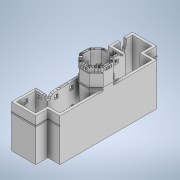
# Autodesk Inventor part: Part1
Saved by Autodesk Inventor 2020 (Build 240168000, 168)
## iProperties
Created: 2021-05-09
Part Number: Part1
Material: Generic
Document SubType Name: Modeling
Designer: Vlasciar
Density: 1 g/cm^3
Appearance: Default
Author: Vlasciar
Autodesk Inventor part; units mm, degrees
ref_plane "YZ Plane" through (0, 0, 0) normal (1, 0, 0) x (0, 1, 0)
ref_plane "XZ Plane" through (0, 0, 0) normal (0, 1, 0) x (-1, 0, 0)
ref_plane "XY Plane" through (0, 0, 0) normal (0, 0, 1) x (1, 0, 0)
sketch "Sketch1" plane through (0, 0, 0) normal (0, 1, 0) x (-1, 0, 0)
  line L0 (-10, -40) -> (10, -40)
  line L1 (10, -40) -> (10, 40)
  line L2 (10, 40) -> (-10, 40)
  line L3 (-10, 40) -> (-10, -40)
  line L4 (-10, -40) -> (10, 40) construction
  line L5 (10, -40) -> (-10, 40) construction
  line L6 (0, 30) -> (20, 30)
  line L7 (20, 30) -> (20, 50)
  line L8 (20, 50) -> (0, 50)
  line L9 (0, 50) -> (0, 30)
  line L10 (0, 30) -> (20, 50) construction
  line L11 (20, 30) -> (0, 50) construction
  line L12 (0, -50) -> (20, -50)
  line L13 (20, -50) -> (20, -30)
  line L14 (20, -30) -> (0, -30)
  line L15 (0, -30) -> (0, -50)
  line L16 (0, -50) -> (20, -30) construction
  line L17 (20, -50) -> (0, -30) construction
  line L18 (10, 4.1421) -> (10, -4.1421)
  line L19 (10, -4.1421) -> (4.1421, -10)
  line L20 (4.1421, -10) -> (-4.1421, -10)
  line L21 (-4.1421, -10) -> (-10, -4.1421)
  line L22 (-10, -4.1421) -> (-10, 4.1421)
  line L23 (-10, 4.1421) -> (-4.1421, 10)
  line L24 (-4.1421, 10) -> (4.1421, 10)
  line L25 (4.1421, 10) -> (10, 4.1421)
  point P0 (0, 0)
  point P1 (0, 0)
  point P2 (10, -40)
  point P3 (0, 40)
  point P4 (0, -40)
  point P5 (10, -30)
  point P6 (10, 30)
  point P7 (-10, -4.1421)
  dimension "d0" = 80
  dimension "d1" = 20
  dimension "d2" = 20
  dimension "d3" = 20
  constraints: 52 end point, 7 midpoint, 6 parallel, 5 perpendicular, 3 horizontal, 1 coincident, 1 point on line, 1 vertical alignment, 17 other
  measures "d0" distance of L0.end L1.end
  measures "d1" distance of L1.end L2.end
  measures "d2" distance of L8.end L7.end
  measures "d3" distance of L14.end L13.end
extrude "Extrusion1" add sketch "Sketch1" along normal blind 32
shell "Shell1" thickness 2 removed faces 1 at (3.3333, 32, 10)
extrude "Extrusion2" add sketch "Sketch1" along normal blind 47 contours L3 L23 L24 L25 L1 L19 L20 L21
sketch "Sketch2" plane through (-20, 0, -50) normal (-1, 0, 0) x (0, 0, 1)
  line L0 (0, 0) -> (20, 0) projected
  line L1 (8, 22) -> (11.5, 22)
  line L2 (11.5, 22) -> (11.5, 12)
  line L3 (11.5, 12) -> (8, 12)
  line L4 (8, 12) -> (8, 22)
  arc A0 (11.5, 22) -> (8, 22) centre (9.75, 17.3163) ccw
  line L5 (12.25, 12) -> (7.25, 12)
  line L6 (7.25, 12) -> (7.25, 22.5633)
  line L7 (12.25, 22.5633) -> (12.25, 12)
  arc A1 (12.25, 22.5633) -> (7.25, 22.5633) centre (9.75, 18.8216) ccw
  line L8 (8.5858, 23.1684) -> (8.5858, 24)
  line L9 (8.5858, 24) -> (9, 24)
  line L10 (9, 24) -> (8, 26)
  line L11 (8, 26) -> (8, 27.1645)
  line L12 (8, 27.1645) -> (7.25, 28.1134)
  line L13 (7.25, 28.1134) -> (7, 32)
  line L14 (12, 32) -> (43.8579, 32) projected
  line L15 (10.6101, 24) -> (10.3293, 23.2842)
  line L16 (7, 32) -> (11.5, 32)
  line L17 (11.5, 32) -> (12.167, 32)
  line L18 (45.8579, 32) -> (10, 32) projected
  line L19 (12.167, 32) -> (12.167, 28.6709)
  line L20 (12, 2) -> (12, 32) projected
  line L21 (12.167, 28.6709) -> (11.5, 27.1645)
  line L22 (11.5, 27.1645) -> (11.3101, 25.7841)
  line L23 (11.3101, 25.7841) -> (10.6101, 24)
  point P0 (50, 0)
  point P1 (12.6775, 32)
  point P2 (8, 12)
  point P3 (11.5, 12)
  point P4 (10.6101, 24)
  point P5 (12, 28.2938)
  dimension "d9" = 12
  dimension "d10" = 10
  dimension "d11" = 3.5
  dimension "d12" = 5
  dimension "d13" = 0.75
  dimension "d14" = 0.75
  dimension "d15" = 4.5
  constraints: 40 end point, 6 point on circle, 5 parallel, 4 point on line, 2 centre point, 2 horizontal, 2 perpendicular, 1 vertical
  measures "d9" distance between parallel lines of L0 L3
  measures "d10" distance of L3.end L1.start
  measures "d11" distance of L2.end L3.end
  measures "d12" radius of A0
  measures "d13" distance between parallel lines of L7 L2
  measures "d14" distance between parallel lines of L6 L4
  measures "d15" radius of A1
extrude "Extrusion3" cut sketch "Sketch2" against normal blind 2 contours A0 L1 | L1 L2 L3 L4
extrude "Extrusion4" cut sketch "Sketch2" against normal blind 1 contours L4 L5 L6 A1 L20 L2 A0 | L20 A1 L7 L5
extrude "Extrusion6" cut sketch "Sketch2" against normal blind 2 contours L8 L9 L10 L11 L12 L13 L16 L17 L20 L21 L22 L23 L15 A1
sketch "Sketch3" plane through (-20, 0, -50) normal (-1, 0, 0) x (0, 0, 1)
  line L0 (0, 0) -> (0, 32) projected
  line L1 (0, 0) -> (20, 0) projected
  line L2 (20, 0) -> (20, 32) projected
  line L3 (11.5, 27.1645) -> (11.3101, 25.7841) projected
  line L4 (11.3101, 25.7841) -> (10.3293, 23.2842) projected
  line L5 (9, 24) -> (8, 26) projected
  line L6 (0, 0) -> (0, 32) projected
  line L7 (0, 25) -> (20, 25)
  line L8 (20, 0) -> (20, 32) projected
  line L9 (0, 26) -> (20, 26)
  point P0 (50, 0)
  point P1 (11.3398, 26)
  point P2 (11.0025, 25)
  point P3 (0, 26)
  point P4 (0, 25)
  point P5 (8.5, 25)
  dimension "d24" = 25
  dimension "d25" = 1
  constraints: 4 end point, 4 point on line, 1 horizontal, 1 perpendicular
  measures "d24" distance between parallel lines of L1 L7
  measures "d25" distance between parallel lines of L9 L7
extrude "Extrusion7" add sketch "Sketch3" along normal blind 0.25 contours L0 L9 L5 L7 | L7 L4 L3 L9 L2
ref_plane "Work Plane1" through (-20.25, 25, -50) normal (0, 1, 0) x (0, 0, 1)
sketch "Sketch4" plane through (-20.25, 25, -50) normal (0, 1, 0) x (0, 0, 1)
  line L0 (20.25, 0) -> (20.25, 10)
  line L1 (20.25, 10) -> (79.75, 10)
  line L2 (79.75, 10) -> (79.75, 0)
  line L3 (79.75, 0) -> (100.25, 0)
  line L4 (100.25, 0) -> (100.25, 20.5)
  line L5 (100.25, 20.5) -> (90.25, 20.5)
  line L6 (90.25, 20.5) -> (90.25, 30.25)
  line L7 (9.75, 30.25) -> (9.75, 20.5)
  line L8 (9.75, 20.5) -> (-0.25, 20.5)
  line L9 (-0.25, 20.5) -> (-0.25, 0)
  line L10 (8, 0) -> (0, 0) projected
  line L11 (-0.25, 0) -> (0, 0)
  line L12 (0, 20.25) -> (0, 0.25) projected
  line L13 (10, 20.25) -> (0, 20.25) projected
  line L14 (10, 30.25) -> (10, 20.25) projected
  line L15 (9.75, 30.25) -> (10, 30.25)
  line L16 (90, 20.25) -> (90, 30.25) projected
  line L17 (90, 30.25) -> (10, 30.25) projected
  line L18 (90, 30.25) -> (90.25, 30.25)
  line L19 (100, 0.25) -> (100, 20.25) projected
  line L20 (80, 10.25) -> (80, 0.25) projected
  line L21 (54.1421, 10.25) -> (80, 10.25) projected
  line L22 (20, 0.25) -> (20, 10.25) projected
  line L23 (20, 0.25) -> (20, 0) projected
  line L24 (20.25, 0) -> (20, 0)
  line L25 (0, 0) -> (20.25, 0)
  line L26 (10, 30.25) -> (90, 30.25)
  line L27 (90, 30.25) -> (90, 20.25)
  line L28 (100, 20.25) -> (90, 20.25)
  line L29 (100, 20.25) -> (100, 0.25)
  line L30 (100, 0.25) -> (80, 0.25)
  line L31 (20, 10.25) -> (80, 10.25) projected
  line L32 (80, 10.25) -> (80, 0.25) projected
  line L33 (80, 10.25) -> (80, 0.25)
  line L34 (80, 10.25) -> (20, 10.25)
  line L35 (20, 10.25) -> (20, 0)
  line L36 (20, 0.25) -> (11.0025, 0.25) projected
  line L37 (0, 0.25) -> (0, 0)
  point P0 (50, 20.25)
  dimension "d28" = 0.25
  dimension "d29" = 0.25
  dimension "d30" = 0.25
  dimension "d31" = 0.25
  dimension "d32" = 0.25
  dimension "d33" = 0.25
  dimension "d34" = 0.25
  dimension "d35" = 0.25
  constraints: 48 end point, 9 perpendicular, 4 collinear, 3 horizontal, 2 point on line, 2 vertical, 1 parallel
  measures "d28" distance between parallel lines of L12 L9
  measures "d29" distance between parallel lines of L13 L8
  measures "d30" distance between parallel lines of L14 L7
  measures "d31" distance between parallel lines of L6 L16
  measures "d32" distance between parallel lines of L4 L19
  measures "d33" distance between parallel lines of L20 L2
  measures "d34" distance between parallel lines of L21 L1
  measures "d35" distance between parallel lines of L22 L0
extrude "Extrusion8" add sketch "Sketch4" along normal blind 1 contours L24 L23 L22 L31 L21 L20 L30 L19 L28 L16 L18 L6 L5 L4 L3 L2 L1 L0
extrude "Extrusion9" add sketch "Sketch4" along normal blind 1 contours L11 L9 L8 L7 L15 L14 L13 L12 L37
sketch "Sketch5" plane through (0, 32, 0) normal (0, 1, 0) x (1, 0, 0)
  line L0 (-10, 30) -> (-10, 4.1421) projected
  line L1 (-10, 4.1421) -> (-8, 6.1421) projected
  line L2 (-8, 6.1421) -> (-8, 32) projected
  line L3 (-10, 30) -> (-8, 30)
  line L4 (-8, 32) -> (-8, 6.1421) projected
  line L5 (-10, 30) -> (-10, -30) projected
  line L6 (-10, -30) -> (-8, -30)
  line L7 (-8, -6.1421) -> (-8, -32) projected
  line L8 (-8, -30) -> (-8, -6.1421)
  line L9 (-10, -4.1421) -> (-4.1421, -10) projected
  line L10 (-10, -4.1421) -> (-10, -30)
  line L11 (-8, -6.1421) -> (-10, -4.1421)
  point P0 (0, 0)
  constraints: 10 end point, 2 parallel, 2 point on line, 1 horizontal, 1 vertical
extrude "Extrusion10" add sketch "Sketch5" along normal blind 2.5
sketch "Sketch6" plane through (-10, 47, -4.1421) normal (-1, 0, 0) x (0, 0, 1)
  line L0 (-25.8579, -47) -> (34.1421, -47) projected
  line L1 (6.0171, -18.8839) -> (2.2671, -18.8839)
  line L2 (2.2671, -18.8839) -> (2.2671, -14.3839)
  line L3 (2.2671, -14.3839) -> (6.0171, -14.3839)
  line L4 (6.0171, -14.3839) -> (6.0171, -18.8839)
  line L5 (6.0171, -18.8839) -> (2.2671, -14.3839) construction
  line L6 (2.2671, -18.8839) -> (6.0171, -14.3839) construction
  line L7 (5.5171, -18.2839) -> (2.7671, -18.2839)
  line L8 (2.7671, -18.2839) -> (2.7671, -14.9839)
  line L9 (2.7671, -14.9839) -> (5.5171, -14.9839)
  line L10 (5.5171, -14.9839) -> (5.5171, -18.2839)
  line L11 (5.5171, -18.2839) -> (2.7671, -14.9839) construction
  line L12 (2.7671, -18.2839) -> (5.5171, -14.9839) construction
  point P0 (4.1421, -47)
  point P1 (4.1421, -16.6339)
  point P2 (4.1421, -47)
  dimension "d42" = 3.75
  dimension "d43" = 4.5
  dimension "d44" = 2.75
  constraints: 24 end point, 5 midpoint, 4 parallel, 2 horizontal, 2 perpendicular, 1 point on line, 1 vertical alignment
  measures "d42" distance of L2.end L3.end
  measures "d43" distance of L1.end L2.end
  measures "d44" distance of L8.end L9.end
extrude "Extrusion11" cut sketch "Sketch6" against normal blind 2.5 contours L7 L8 L9 L10
extrude "Extrusion12" cut sketch "Sketch6" against normal blind 0.5 contours L1 L2 L3 L4 | L7 L8 L9 L10
pattern_linear "Rectangular Pattern1" count 3 spacing 12.5 along (0, 0, 1) count 2 spacing 14 along (0, -1, 0) of "Extrusion12", "Extrusion11"
pattern_linear "Rectangular Pattern2" count 3 spacing 12.5 along (0, 0, -1) count 2 spacing 14 along (0, -1, 0) of "Extrusion12", "Extrusion11"
sketch "Sketch7" plane through (-10, 47, -4.1421) normal (-1, 0, 0) x (0, 0, 1)
  line L0 (-25.8579, -12.5) -> (0, -12.5) projected
  line L1 (-25.8579, -15) -> (-25.8579, -12.5) projected
  line L2 (-25.8579, -15) -> (-24.9155, -14.8512)
  line L3 (-24.9155, -14.8512) -> (-24.7999, -14.2836)
  line L4 (-24.7999, -14.2836) -> (-23.2973, -13.787)
  line L5 (-23.2973, -13.787) -> (-22.7637, -12.9023)
  line L6 (-22.7637, -12.9023) -> (-22.5613, -12.5)
  line L7 (-22.5613, -12.5) -> (-19.8497, -12.5)
  line L8 (-19.8497, -12.5) -> (-17.8318, -13.1696)
  line L9 (-13.0388, -13.2248) -> (-11.5153, -12.5)
  line L10 (-11.5153, -12.5) -> (-9.0025, -12.5874)
  line L11 (-9.0025, -12.5874) -> (-6.8279, -12.5)
  line L12 (-6.8279, -12.5) -> (-5.8631, -12.6965)
  line L13 (-2.1188, -13.2003) -> (-1.5625, -13.178)
  line L14 (-1.5625, -13.178) -> (-0.4501, -12.6488)
  line L15 (-0.4501, -12.6488) -> (0, -12.5)
  line L16 (-17.8318, -13.1696) -> (-15.3761, -13.3447)
  line L17 (-15.3761, -13.3447) -> (-12.9874, -13.2003)
  line L18 (-5.8631, -12.6965) -> (-3.9239, -12.8348)
  line L19 (-3.9239, -12.8348) -> (-2.1188, -13.2003)
  point P0 (4.1421, -47)
  constraints: 36 end point, 7 point on line, 4 parallel
extrude "Extrusion13" cut sketch "Sketch7" against normal up to surface (2 mm away)
pattern_linear "Rectangular Pattern3" count 2 spacing 9 along (0, 1, 0) of "Extrusion11", "Extrusion12"
sketch "Sketch8" plane through (0, 47, 0) normal (0, 1, 0) x (1, 0, 0)
  line L0 (10, -4.1421) -> (10, 4.1421) projected
  line L1 (8, 3.3137) -> (8, -3.3137)
  line L2 (8, -3.3137) -> (3.3137, -8)
  line L3 (3.3137, -8) -> (-3.3137, -8)
  line L4 (-3.3137, -8) -> (-8, -3.3137)
  line L5 (-8, -3.3137) -> (-8, 3.3137)
  line L6 (-8, 3.3137) -> (-3.3137, 8)
  line L7 (-3.3137, 8) -> (3.3137, 8)
  line L8 (3.3137, 8) -> (8, 3.3137)
  point P0 (0, 0)
  point P1 (0, 0)
  dimension "d66" = 2
  dimension "d67" = 2
  constraints: 16 end point, 1 coincident, 17 other
  measures "d66" distance from line of L0 L1.start
  measures "d67" distance from line of L0 L1.end
extrude "Extrusion14" cut sketch "Sketch8" against normal blind 45
sketch "Sketch9" plane through (-10, 47, -4.1421) normal (-1, 0, 0) x (0, 0, 1)
  line L0 (8.2843, -12.5) -> (34.1421, -12.5) projected
  line L1 (8.2843, -12.5) -> (8.2843, 0) projected
  line L2 (0, -12.5) -> (0, 0) projected
  line L3 (8.2843, -12.5) -> (10.2843, -12.5) projected
  line L4 (8.4943, -12.5) -> (-0.21, -12.5)
  line L5 (-0.21, -12.5) -> (-0.21, -11.5)
  line L6 (-0.21, -11.5) -> (8.4943, -11.5)
  line L7 (8.4943, -11.5) -> (8.4943, -12.5)
  line L8 (-0.21, -12.1053) -> (8.4943, -12.1053)
  line L9 (8.4943, -12.1053) -> (8.4292, -12.1053)
  line L10 (8.4943, -12.5) -> (8.2843, -12.5)
  line L11 (8.2843, -12.5) -> (8.2843, -12.1053)
  line L12 (8.2843, -12.1053) -> (8.4943, -12.1053)
  line L13 (8.4943, -12.1053) -> (8.4943, -12.5)
  point P0 (4.1421, -47)
  point P1 (8.2843, -12.5)
  dimension "d70" = 0.21
  dimension "d71" = 0.21
  dimension "d72" = 1
  constraints: 20 end point, 6 point on line, 4 parallel, 3 perpendicular, 2 horizontal
  measures "d70" distance between parallel lines of L2 L5
  measures "d71" distance between parallel lines of L7 L1
  measures "d72" distance between parallel lines of L6 L4
extrude "Extrusion15" add sketch "Sketch9" along normal blind 0.5
pattern_circular "Circular Pattern1" count 8 over 360 about axis through (0, -10, 0) along (0, 1, 0) of "Extrusion15"
pattern_linear "Rectangular Pattern4" count 2 spacing 9 along (0, 1, 0) of "Extrusion15", "Circular Pattern1"
sketch "Sketch10" plane through (-10, 47, -4.1421) normal (-1, 0, 0) x (0, 0, 1)
  line L0 (0, -2.5) -> (8.2843, -2.5) projected
  line L1 (0, 0) -> (8.2843, 0) projected
  line L2 (7.4558, 0) -> (0.8284, 0) projected
  line L3 (4.9026, -2.5) -> (3.3817, -2.5)
  line L4 (3.3817, -2.5) -> (3.3817, -0.5122)
  line L5 (4.9026, -0.5122) -> (4.9026, -2.5)
  arc A0 (4.9026, -0.5122) -> (3.3817, -0.5122) centre (4.1421, -1.1616) ccw
  arc A1 (6.9026, -0.5122) -> (5.3817, -0.5122) centre (6.1421, -1.1616) ccw
  line L6 (6.9026, -0.5122) -> (6.9026, -2.5)
  line L7 (5.3817, -2.5) -> (5.3817, -0.5122)
  line L8 (6.9026, -2.5) -> (5.3817, -2.5)
  arc A2 (2.9026, -0.5122) -> (1.3817, -0.5122) centre (2.1421, -1.1616) ccw
  line L9 (2.9026, -0.5122) -> (2.9026, -2.5)
  line L10 (2.9026, -2.5) -> (1.3817, -2.5)
  line L11 (1.3817, -2.5) -> (1.3817, -0.5122)
  point P0 (4.1421, -47)
  point P1 (4.1421, -1.25)
  dimension "d81" = 1
  dimension "d84" = 2
  dimension "d91" = 2
  constraints: 18 end point, 6 point on circle, 3 centre point, 3 horizontal, 1 parallel, 1 perpendicular, 18 other
  measures "d81" radius of A0
  measures "d84" distance of A0.centre A1.centre
  measures "d91" distance of A0.centre A2.centre
extrude "Extrusion16" cut sketch "Sketch10" against normal blind 0.5
pattern_circular "Circular Pattern2" count 8 over 360 about axis through (0, -10, 0) along (0, 1, 0) of "Extrusion16"
sketch "Sketch11" plane through (0, 47, 0) normal (0, 1, 0) x (1, 0, 0)
  line L0 (-8, 3.3137) -> (-3.3137, 8) projected
  line L1 (-3.3137, 8) -> (3.3137, 8) projected
  line L2 (3.3137, 8) -> (8, 3.3137) projected
  line L3 (8, 3.3137) -> (8, -3.3137) projected
  line L4 (8, -3.3137) -> (3.3137, -8) projected
  line L5 (3.3137, -8) -> (-3.3137, -8) projected
  line L6 (-3.3137, -8) -> (-8, -3.3137) projected
  line L7 (-8, -3.3137) -> (-8, 3.3137) projected
  line L8 (-4.1421, 10) -> (-10, 4.1421) projected
  line L9 (-10, 4.1421) -> (-10, -4.1421) projected
  line L10 (-10, -4.1421) -> (-4.1421, -10) projected
  line L11 (-4.1421, -10) -> (4.1421, -10) projected
  line L12 (4.1421, -10) -> (10, -4.1421) projected
  line L13 (10, -4.1421) -> (10, 4.1421) projected
  line L14 (10, 4.1421) -> (4.1421, 10) projected
  line L15 (4.1421, 10) -> (-4.1421, 10) projected
  point P0 (0, 0)
extrude "Extrusion17" add sketch "Sketch11" along normal blind 1
sketch "Sketch12" plane through (-10, 44.5, 2.7605) normal (-1, 0, 0) x (0, 0, 1)
  line L0 (1.3817, 0) -> (1.3817, 3.5) projected
  line L1 (-6.9026, 3.5) -> (1.3817, 3.5) projected
  line L2 (-6.9026, 0) -> (-6.9026, 3.5) projected
  line L3 (1.3817, 0) -> (1.3817, 3.5) projected
  line L4 (1.3817, 3.0258) -> (-6.9026, 3.0258)
  line L5 (1.3817, 3.0258) -> (0.7961, 3.2794)
  line L6 (0.7961, 3.2794) -> (0.4566, 3.2083)
  line L7 (0.4566, 3.2083) -> (0.2925, 3.2794)
  line L8 (0.2925, 3.2794) -> (-0.1751, 3.3426)
  line L9 (-0.1751, 3.3426) -> (-0.2698, 3.2794)
  line L10 (-0.2698, 3.2794) -> (-0.5516, 3.2204)
  line L11 (-0.5516, 3.2204) -> (-1.0436, 3.2204)
  line L12 (-1.0436, 3.2204) -> (-1.3256, 3.3426)
  line L13 (-1.3256, 3.3426) -> (-1.5269, 3.2083)
  line L14 (-1.5269, 3.2083) -> (-1.8368, 3.3426)
  line L15 (-1.8368, 3.3426) -> (-2.2547, 3.399)
  line L16 (-2.2547, 3.399) -> (-2.628, 3.4494)
  line L17 (-2.628, 3.4494) -> (-2.9564, 3.3976)
  line L18 (-2.9564, 3.3976) -> (-3.395, 3.2204)
  line L19 (-3.395, 3.2204) -> (-3.8024, 3.2755)
  line L20 (-3.8024, 3.2755) -> (-4.2992, 3.3426)
  line L21 (-4.2992, 3.3426) -> (-4.7605, 3.3426)
  line L22 (-6.0742, 3.5) -> (0.5532, 3.5) projected
  line L23 (-4.7605, 3.3426) -> (-5.289, 3.2319)
  line L24 (-5.289, 3.2319) -> (-5.6985, 3.2873)
  line L25 (-5.6985, 3.2873) -> (-6.4207, 3.2204)
  line L26 (-6.4207, 3.2204) -> (-6.9026, 3.0258)
  point P0 (-2.7605, -44.5)
  constraints: 44 end point, 12 parallel, 6 point on line, 1 horizontal
extrude "Extrusion18" cut sketch "Sketch12" against normal blind 2 contours L5 L6 L7 L8 L9 L10 L11 L12 L13 L14 L15 L16 L17 L18 L19 L20 L21 L23 L24 L25 L26 L2 L1 L0
pattern_circular "Circular Pattern3" count 8 over 360 about axis through (0, -10, 0) along (0, 1, 0) of "Extrusion18"
sketch "Sketch13" plane through (-10, 35.5, -4.1421) normal (-1, 0, 0) x (0, 0, 1)
  line L0 (8.2843, 8) -> (0, 8) projected
  line L1 (0, 0) -> (0, 8) projected
  line L2 (8.2843, 0) -> (8.2843, 8) projected
  line L3 (2.2671, 1.6161) -> (2.2671, 6.1161) projected
  line L4 (2.2671, 6.1161) -> (6.0171, 6.1161) projected
  line L5 (6.0171, 6.1161) -> (6.0171, 1.6161) projected
  line L6 (1.9172, 6.1161) -> (6.3671, 6.1161)
  line L7 (6.3671, 6.1161) -> (4.1343, 8)
  line L8 (1.9172, 6.1161) -> (4.1343, 8)
  line L9 (1.9172, 6.1161) -> (6.3671, 6.1161)
  line L10 (6.3671, 6.1161) -> (4.1343, 8)
  line L11 (1.9172, 6.1161) -> (4.1343, 8)
  line L12 (6.0408, 6.2532) -> (4.1343, 7.8617)
  line L13 (2.2412, 6.2532) -> (6.0408, 6.2532)
  line L14 (2.2412, 6.2532) -> (4.1343, 7.8617)
  point P0 (4.1421, -35.5)
  point P1 (2.2671, 6.1161)
  point P2 (6.0171, 6.1161)
  dimension "d108" = 0.3499
  dimension "d109" = 0.35
  dimension "d110" = 4.15
  dimension "d111" = 4.1343
  constraints: 18 end point, 2 point on line, 1 horizontal
  measures "d108" distance from line of L3 L6.start
  measures "d109" distance from line of L5 L6.end
  measures "d110" distance from line of L7.end L2
  measures "d111" distance from line of L1 L7.end
extrude "Extrusion19" add sketch "Sketch13" along normal blind 0.5 contours L6 L8 L7 L4 | L13 L14 L12
extrude "Extrusion20" cut sketch "Sketch9" along normal blind 0.5 contours L1 L8 L7 L0 | L4 L2 L8 L1 | L4 L5 L8 L2
extrude "Extrusion21" add sketch "Sketch9" along normal blind 0.25 contours L1 L8 L7 L0 | L4 L2 L8 L1 | L4 L5 L8 L2
pattern_circular "Circular Pattern4" count 8 over 360 about axis through (0, -10, 0) along (0, 1, 0) of "Extrusion21", "Extrusion20"
pattern_linear "Rectangular Pattern5" count 2 spacing 9 along (0, 1, 0) of "Extrusion20", "Extrusion21", "Circular Pattern4"
extrude "Extrusion22" cut sketch "Sketch13" along normal blind 5 contours L13 L14 L12
extrude "Extrusion23" add sketch "Sketch13" along normal blind 0.25 contours L13 L14 L12
pattern_linear "Rectangular Pattern6" count 2 spacing 9 along (0, -1, 0) of "Extrusion22", "Extrusion23", "Extrusion19"
pattern_linear "Rectangular Pattern7" count 2 spacing 23 along (0, -1, 0) of "Extrusion23", "Extrusion22", "Extrusion19"
sketch "Sketch14" plane through (-10, 0, -30) normal (-1, 0, 0) x (0, 0, 1)
  line L0 (30, 0) -> (25.5, 0)
  line L1 (25.5, 0) -> (25.5, 9)
  line L2 (25.5, 9) -> (30, 9)
  line L3 (30, 9) -> (30, 0)
  arc A0 (30, 9) -> (25.5, 5.0081) centre (30.4006, 4.0161) ccw
  line L4 (60, 0) -> (0, 0)
  line L5 (34.5, 0) -> (34.5, 9)
  line L6 (34.5, 9) -> (30, 9)
  arc A1 (34.5, 5.0081) -> (30, 9) centre (29.5994, 4.0161) ccw
  line L7 (25.5, 0) -> (24.5, 0)
  line L8 (24.5, 0) -> (24.5, 9)
  line L9 (24.5, 9) -> (25.5, 9)
  line L10 (25.5, 9) -> (25.5, 0)
  line L11 (34.5, 0) -> (35.5, 0)
  line L12 (35.5, 0) -> (35.5, 9)
  line L13 (35.5, 9) -> (34.5, 9)
  line L14 (34.5, 9) -> (34.5, 0)
  line L15 (23.8579, 33.8044) -> (23.8579, 2) projected
  line L16 (23.8579, 10.273) -> (36.0712, 10.273)
  line L17 (36.0712, 10.273) -> (29.8579, 13.773)
  line L18 (29.8579, 13.773) -> (23.8579, 10.273)
  line L19 (34.8884, 10.5726) -> (29.8579, 13.4063)
  line L20 (25, 10.5726) -> (34.8884, 10.5726)
  line L21 (29.8579, 13.4063) -> (25, 10.5726)
  point P0 (24.5, 0)
  dimension "d134" = 4.5
  dimension "d135" = 9
  dimension "d137" = 5
  dimension "d138" = 1
  dimension "d139" = 1
  dimension "d140" = 3.5
  dimension "d141" = 6
  constraints: 42 end point, 7 parallel, 6 symmetric about line, 4 horizontal, 4 point on circle, 4 point on line, 3 perpendicular, 2 centre point, 1 other
  measures "d134" distance of L1.end L2.end
  measures "d135" distance of L0.end L1.end
  measures "d137" radius of A0
  measures "d138" distance of L8.end L9.end
  measures "d139" distance of L12.end L13.end
  measures "d140" distance from line of L16 L17.end
  measures "d141" distance from line of L15 L17.end
extrude "Extrusion24" add sketch "Sketch14" along normal blind 0.25 contours A0 L1 L2 | L6 L5 A1 | L20 L21 L19
extrude "Extrusion25" add sketch "Sketch14" along normal blind 0.5 contours L18 L17 L16
extrude "Extrusion26" add sketch "Sketch14" along normal blind 0.75 contours L4 L8 L9 L1 | L5 L13 L12 L4
extrude "Extrusion27" cut sketch "Sketch14" against normal blind 2 contours L0 L1 A0 L3 | L3 A1 L5 L4
sketch "Sketch15" plane through (0, 0, 0) normal (0, -1, 0) x (1, 0, 0)
  line L0 (-8, -4.5) -> (-10.75, -4.5) projected
  line L1 (-10.75, -5.5) -> (-10.75, -4.5) projected
  line L2 (-10, -5.5) -> (-10.75, -5.5) projected
  line L3 (-10, -30) -> (-10, -5.5) projected
  line L4 (-20, -30) -> (-10, -30) projected
  line L5 (-20, -50) -> (-20, -30) projected
  line L6 (0, -50) -> (-20, -50) projected
  line L7 (0, -40) -> (0, -50) projected
  line L8 (10, -40) -> (0, -40) projected
  line L9 (10, 40) -> (10, -40) projected
  line L10 (0, 40) -> (10, 40) projected
  line L11 (0, 50) -> (0, 40) projected
  line L12 (-20, 50) -> (0, 50) projected
  line L13 (-20, 30) -> (-20, 50) projected
  line L14 (-10, 30) -> (-20, 30) projected
  line L15 (-10, 5.5) -> (-10, 30) projected
  line L16 (-10, 5.5) -> (-10.75, 5.5) projected
  line L17 (-10.75, 4.5) -> (-10.75, 5.5) projected
  line L18 (-10.75, 4.5) -> (-8, 4.5) projected
  line L19 (-8, 4.5) -> (-8, -4.5) projected
  point P0 (0, 0)
extrude "Extrusion28" add sketch "Sketch15" along normal blind 2
sketch "Sketch16" plane through (-18, 2, 48) normal (0, 1, 0) x (1, 0, 0)
  line L0 (13.8579, 38) -> (10, 41.8579) projected
  line L1 (10, 41.8579) -> (10, 16) projected
  line L2 (10, 16) -> (0, 16) projected
  line L3 (0, 16) -> (0, 0) projected
  line L4 (0, 0) -> (16, 0) projected
  line L5 (16, 0) -> (16, 10) projected
  line L6 (16, 10) -> (26, 10) projected
  line L7 (26, 10) -> (26, 41.8579) projected
  line L8 (26, 41.8579) -> (22.1421, 38) projected
  line L9 (22.1421, 38) -> (13.8579, 38) projected
  point P0 (18, 48)
sketch "Sketch17" plane through (0, 2, 0) normal (0, 1, 0) x (1, 0, 0)
  line L0 (-8, 3.3137) -> (-3.3137, 8) projected
  line L1 (-8, -3.3137) -> (-8, 3.3137) projected
  line L2 (-3.3137, -8) -> (-8, -3.3137) projected
  line L3 (3.3137, -8) -> (-3.3137, -8) projected
  line L4 (8, -3.3137) -> (3.3137, -8) projected
  line L5 (8, 3.3137) -> (8, -3.3137) projected
  line L6 (3.3137, 8) -> (8, 3.3137) projected
  line L7 (-3.3137, 8) -> (3.3137, 8) projected
  point P0 (0, 0)
sketch "Sketch18" plane through (-18, 2, -48) normal (0, 1, 0) x (1, 0, 0)
  line L0 (10, -41.8579) -> (13.8579, -38) projected
  line L1 (13.8579, -38) -> (22.1421, -38) projected
  line L2 (22.1421, -38) -> (26, -41.8579) projected
  line L3 (26, -41.8579) -> (26, -10) projected
  line L4 (26, -10) -> (16, -10) projected
  line L5 (16, -10) -> (16, 0) projected
  line L6 (16, 0) -> (0, 0) projected
  line L7 (0, 0) -> (0, -16) projected
  line L8 (0, -16) -> (10, -16) projected
  line L9 (10, -16) -> (10, -41.8579) projected
  point P0 (18, -48)
extrude "Extrusion29" cut sketch "Sketch18" against normal blind 2
extrude "Extrusion30" cut sketch "Sketch17" against normal blind 2
extrude "Extrusion31" cut sketch "Sketch16" against normal blind 2
sketch "Sketch19" plane through (-8, 0, -30) normal (-1, 0, 0) x (0, 0, 1)
  line L0 (33.3137, 7.3633) -> (33.3137, 0) projected
  line L1 (33.3137, 0) -> (26.6863, 0) projected
  line L2 (26.6863, 7.3633) -> (26.6863, 0) projected
  arc A0 (26.6863, 7.3633) -> (25.5, 5.0081) centre (30.4006, 4.0161) ccw projected
  line L3 (25.5, -2) -> (25.5, 5.0081) projected
  line L4 (34.5, -2) -> (25.5, -2) projected
  line L5 (34.5, 5.0081) -> (34.5, -2) projected
  arc A1 (34.5, 5.0081) -> (33.3137, 7.3633) centre (29.5994, 4.0161) ccw projected
  line L6 (25.5, -1.0006) -> (34.5, -1.0006)
  line L7 (34.5, -1.0006) -> (34.5, -2)
  line L8 (34.5, -2) -> (25.5, -2)
  line L9 (25.5, -2) -> (25.5, -1.0006)
  point P0 (30, 0)
  constraints: 8 end point, 2 parallel, 1 horizontal, 1 perpendicular, 1 point on line
sketch "Sketch20" plane through (-10.25, 9, 4.5) normal (0, 0, -1) x (-1, 0, 0)
  line L0 (-2.25, -3.9919) -> (-2.25, -11) projected
  line L1 (0.5, -11) -> (-2.25, -11) projected
  line L2 (0.5, 0) -> (0.5, -11) projected
  line L3 (-2.25, -9.5) -> (-1.25, -9.5)
  line L4 (-1.25, -9.5) -> (-1.25, -10)
  line L5 (-1.25, -10) -> (-0.25, -10)
  line L6 (-0.25, -10) -> (-0.25, -10.5)
  line L7 (-0.25, -10.5) -> (0.75, -10.5)
  line L8 (-2.25, -9) -> (-6.1079, -9) projected
  line L9 (0.5, 0) -> (0.5, -11) projected
  line L10 (0.5, -10.5) -> (0.5, -11)
  line L11 (0.5, -11) -> (-2.25, -11)
  point P0 (-10.25, -9)
  dimension "d158" = 0.5
  dimension "d159" = 1
  dimension "d160" = 0.5
  dimension "d161" = 1
  dimension "d162" = 0.5
  dimension "d163" = 1
  constraints: 14 end point, 5 perpendicular, 3 point on line, 1 collinear, 1 horizontal
  measures "d158" distance from line of L8 L3.start
  measures "d159" distance of L3.start L3.end
  measures "d160" distance of L3.end L4.end
  measures "d161" distance of L4.end L5.end
  measures "d162" distance of L5.end L6.end
  measures "d163" distance of L6.end L7.end
extrude "Extrusion32" add sketch "Sketch20" along normal up to surface (9 mm away)
sketch "Sketch21" plane through (-10, 26, -30) normal (-1, 0, 0) x (0, 0, 1)
  line L0 (60, 6) -> (60, 8.5) projected
  line L1 (34.4957, 8.5) -> (60, 8.5) projected
  line L2 (60, 6) -> (60, 8.5) projected
  line L3 (60, 7.25) -> (58.4422, 7.428)
  line L4 (58.4422, 7.428) -> (58.0512, 7.8855)
  line L5 (58.0512, 7.8855) -> (56.3953, 8.1528)
  line L6 (56.3953, 8.1528) -> (54.8144, 8.1528)
  line L7 (54.8144, 8.1528) -> (53.4872, 8.1528)
  line L8 (53.4872, 8.1528) -> (53.2121, 8.2912)
  line L9 (53.2121, 8.2912) -> (51.4558, 8.2912)
  line L10 (60, 8.5) -> (36.4957, 8.5) projected
  line L11 (51.4558, 8.2912) -> (51.1024, 8.1748)
  line L12 (51.1024, 8.1748) -> (50.531, 8.2912)
  line L13 (50.531, 8.2912) -> (49.301, 8.2912)
  line L14 (49.301, 8.2912) -> (48.2975, 8.3351)
  line L15 (48.2975, 8.3351) -> (47.0466, 8.2912)
  line L16 (47.0466, 8.2912) -> (46.0903, 8.2912)
  line L17 (46.0903, 8.2912) -> (45.1224, 8.3336)
  line L18 (45.1224, 8.3336) -> (44.216, 8.2912)
  line L19 (44.216, 8.2912) -> (42.9402, 8.3471)
  line L20 (42.9402, 8.3471) -> (41.6575, 8.4032)
  line L21 (41.6575, 8.4032) -> (40.3035, 8.5)
  line L22 (58.4422, 7.428) -> (59.4222, 6.2814)
  line L23 (59.4222, 6.2814) -> (60, 4.5272)
  line L24 (60, 0) -> (60, 6) projected
  point P0 (30, -26)
  constraints: 40 end point, 9 point on line, 3 parallel, 1 horizontal, 1 midpoint
extrude "Extrusion33" cut sketch "Sketch21" against normal blind 2 contours L3 L4 L5 L6 L7 L8 L9 L11 L12 L13 L14 L15 L16 L17 L18 L19 L20 L21 L1 L0
sketch "Sketch23" plane through (0, 32, 0) normal (0, 1, 0) x (1, 0, 0)
  line L0 (-8, -30) -> (-10, -30) projected
  line L1 (-10, -30) -> (-20, -30) projected
  line L2 (-20, -30) -> (-20, -50) projected
  line L3 (-20, -50) -> (0, -50) projected
  line L4 (0, -50) -> (0, -40) projected
  line L5 (0, -40) -> (10, -40) projected
  line L6 (10, -40) -> (10, -4.1421) projected
  line L7 (10, -4.1421) -> (8, -6.1421) projected
  line L8 (8, -6.1421) -> (8, -38) projected
  line L9 (8, -38) -> (-2, -38) projected
  line L10 (-2, -38) -> (-2, -48) projected
  line L11 (-2, -48) -> (-18, -48) projected
  line L12 (-18, -48) -> (-18, -32) projected
  line L13 (-18, -32) -> (-8, -32) projected
  line L14 (-8, -32) -> (-8, -30) projected
  point P0 (0, 0)
extrude "Extrusion34" add sketch "Sketch23" along normal blind 1
sketch "Sketch24" plane through (0, 32, 0) normal (0, 1, 0) x (1, 0, 0)
  line L0 (-20, 43) -> (-18, 43) projected
  line L1 (-18, 43) -> (-18, 48) projected
  line L2 (-18, 48) -> (-2, 48) projected
  line L3 (-2, 48) -> (-2, 38) projected
  line L4 (-2, 38) -> (8, 38) projected
  line L5 (8, 38) -> (8, 6.1421) projected
  line L6 (8, 6.1421) -> (10, 4.1421) projected
  line L7 (10, 4.1421) -> (10, 40) projected
  line L8 (10, 40) -> (0, 40) projected
  line L9 (0, 40) -> (0, 50) projected
  line L10 (0, 50) -> (-20, 50) projected
  line L11 (-20, 50) -> (-20, 43) projected
  point P0 (0, 0)
extrude "Extrusion35" add sketch "Sketch24" along normal blind 1
sketch "Sketch25" plane through (-20, 26, 30) normal (-1, 0, 0) x (0, 0, 1)
  line L0 (0, 0) -> (0, 7) projected
  line L1 (-6.875, 6.6161) -> (-3.125, 6.6161) projected
  line L2 (-3.125, 6.6161) -> (-3.125, 2.1161) projected
  line L3 (8.299, 5.7472) -> (12.0034, 5.7472)
  line L4 (12.0034, 5.7472) -> (12.0034, 1.2472)
  line L5 (12.0034, 1.2472) -> (8.299, 1.2472)
  line L6 (8.299, 1.2472) -> (8.299, 5.7472)
  line L7 (-6.375, 2.7161) -> (-6.375, 6.0161) projected
  line L8 (11.5034, 1.8472) -> (8.799, 1.8472)
  line L9 (8.799, 1.8472) -> (8.799, 5.1472)
  line L10 (8.799, 5.1472) -> (11.5034, 5.1472)
  line L11 (11.5034, 5.1472) -> (11.5034, 1.8472)
  line L12 (8.299, -11.7528) -> (8.299, -7.2528)
  line L13 (8.799, -11.1528) -> (8.799, -7.8528)
  line L14 (11.5034, -11.1528) -> (8.799, -11.1528)
  line L15 (8.799, -7.8528) -> (11.5034, -7.8528)
  line L16 (11.5034, -7.8528) -> (11.5034, -11.1528)
  line L17 (8.299, -7.2528) -> (12.0034, -7.2528)
  line L18 (12.0034, -7.2528) -> (12.0034, -11.7528)
  line L19 (12.0034, -11.7528) -> (8.299, -11.7528)
  point P0 (-30, -26)
  point P1 (-3.625, 2.7161)
  point P2 (-5, 4.3661)
  dimension "d174" = 13
  constraints: 24 end point, 4 parallel, 2 horizontal, 2 perpendicular, 1 vertical, 16 other
  measures "d174" distance of L5.end L12.start
extrude "Extrusion36" cut sketch "Sketch25" against normal blind 2 contours L8 L9 L10 L11 | L13 L15 L16 L14
extrude "Extrusion37" cut sketch "Sketch25" against normal blind 0.5 contours L3 L4 L5 L6 | L12 L17 L18 L19 | L13 L15 L16 L14
sketch "Sketch26" plane through (-10, 25, -30) normal (-1, 0, 0) x (0, 0, 1)
  line L0 (19.375, -10.8839) -> (15.625, -10.8839) projected
  line L1 (19.375, -25) -> (15.625, -25)
  line L2 (15.625, -25) -> (15.625, -16.5009)
  line L3 (15.625, -16.5009) -> (19.375, -16.5009)
  line L4 (19.375, -16.5009) -> (19.375, -25)
  arc A0 (30, -16) -> (26.6863, -17.6367) centre (30.4006, -20.9839) ccw projected
  line L5 (6.0142, -17.4077) -> (9.5269, -17.4077)
  line L6 (9.5269, -17.4077) -> (9.5269, -21.5)
  line L7 (9.5269, -21.5) -> (6.0142, -21.5)
  line L8 (6.0142, -21.5) -> (6.0142, -17.4077)
  line L9 (40.625, -17.4077) -> (44.375, -17.4077)
  line L10 (44.375, -17.4077) -> (44.375, -21.4077)
  line L11 (44.375, -21.4077) -> (40.625, -21.4077)
  line L12 (40.625, -21.4077) -> (40.625, -17.4077)
  line L13 (53.125, -17.4077) -> (56.875, -17.4077)
  line L14 (56.875, -17.4077) -> (56.875, -21.4077)
  line L15 (56.875, -21.4077) -> (53.125, -21.4077)
  line L16 (53.125, -21.4077) -> (53.125, -17.4077)
  line L17 (56.375, -21.0577) -> (53.625, -21.0577)
  line L18 (53.625, -21.0577) -> (53.625, -17.7577)
  line L19 (53.625, -17.7577) -> (56.375, -17.7577)
  line L20 (56.375, -17.7577) -> (56.375, -21.0577)
  line L21 (43.875, -21.0577) -> (41.125, -21.0577)
  line L22 (41.125, -21.0577) -> (41.125, -17.7577)
  line L23 (41.125, -17.7577) -> (43.875, -17.7577)
  line L24 (43.875, -17.7577) -> (43.875, -21.0577)
  point P0 (30, -25)
  point P1 (28.1864, -16.5009)
  point P2 (40.625, -6.3839)
  point P3 (44.375, -10.8839)
  point P4 (53.125, -10.8839)
  point P5 (56.875, -10.8839)
  point P6 (42.5, -17.4077)
  point P7 (53.625, -10.2839)
  point P8 (56.375, -10.2839)
  point P9 (43.875, -10.2839)
  point P10 (41.125, -10.2839)
  dimension "d185" = 4
  dimension "d186" = 3.3
  dimension "d187" = 3.3
  dimension "d188" = 0.35
  constraints: 48 end point, 13 parallel, 8 vertical alignment, 6 horizontal, 6 perpendicular, 5 horizontal alignment, 1 midpoint, 1 point on circle, 1 point on line
  measures "d185" distance between parallel lines of L9 L11
  measures "d186" distance between parallel lines of L19 L17
  measures "d187" distance between parallel lines of L23 L21
  measures "d188" distance between parallel lines of L11 L21
extrude "Extrusion38" cut sketch "Sketch26" against normal blind 2 contours L1 L2 L3 L4 | L5 L6 L7 L8
extrude "Extrusion39" cut sketch "Sketch26" against normal blind 2 contours L9 L10 L11 L12 | L13 L14 L15 L16 | L17 L18 L19 L20 | L21 L22 L23 L24
fillet "Fillet1" radius 0.5 12 edges at (-10, 5.5462, -23.9858) (-10, 7.5923, -22.2294) (-10, 5.5462, -20.4731) (-10, 3.5, -22.2294) (-10, 5.5923, 14.375) (-10, 3.5923, 12.5) (-10, 5.5923, 10.625) (-10, 7.5923, 12.5) (-10, 5.5923, 23.125) (-10, 7.5923, 25) (-10, 5.5923, 26.875) (-10, 3.5923, 25)
extrude "Extrusion40" cut sketch "Sketch21" against normal blind 2 contours L24 L23 L22 L3 L0
sketch "Sketch27" plane through (-10, 25, 30) normal (0, 0, -1) x (-1, 0, 0)
  line L0 (6.5282, -10.7156) -> (3.0282, -10.7156)
  line L1 (3.0282, -10.7156) -> (3.0282, -6.7156)
  line L2 (3.0282, -6.7156) -> (6.5282, -6.7156)
  line L3 (6.5282, -6.7156) -> (6.5282, -10.7156)
  line L4 (6.5282, -10.7156) -> (3.0282, -6.7156) construction
  line L5 (3.0282, -10.7156) -> (6.5282, -6.7156) construction
  arc A0 (6.5282, -6.7156) -> (3.0282, -6.7156) centre (4.7782, -9.1523) ccw
  line L6 (6.245, -10.3921) -> (3.3418, -10.3921)
  line L7 (3.3418, -10.3921) -> (3.3418, -7.074)
  line L8 (3.3418, -7.074) -> (6.245, -7.074)
  line L9 (6.245, -7.074) -> (6.245, -10.3921)
  arc A1 (6.245, -7.074) -> (3.3418, -7.074) centre (4.7934, -8.7864) ccw
  line L10 (6.5282, 3.3134) -> (3.0282, 3.3134)
  line L11 (3.0282, 3.3134) -> (3.0282, 6.6956)
  line L12 (3.0282, 6.6956) -> (6.5282, 6.6956)
  line L13 (6.5282, 6.6956) -> (6.5282, 3.3134)
  line L14 (6.0037, 3.7245) -> (3.4869, 3.7245)
  line L15 (3.4869, 3.7245) -> (3.4869, 6.2078)
  line L16 (3.4869, 6.2078) -> (6.0037, 6.2078)
  line L17 (6.0037, 6.2078) -> (6.0037, 3.7245)
  point P0 (-10, -25)
  point P1 (4.7782, -8.7156)
  dimension "d194" = 4
  dimension "d195" = 3.5
  dimension "d196" = 3
  constraints: 36 end point, 8 parallel, 4 horizontal, 4 perpendicular, 4 point on circle, 3 point on line, 2 centre point, 2 midpoint
  measures "d194" distance of L2.end L0.start
  measures "d195" distance of L1.end L2.end
  measures "d196" radius of A0
extrude "Extrusion41" cut sketch "Sketch27" along normal blind 0.5 contours L0 L1 L2 A1 L7 L6 L9 L3 | L2 A1 A0
extrude "Extrusion42" cut sketch "Sketch27" against normal blind 2 contours A1 L8 L2 | L2 A1 | L9 L6 L7 L8
extrude "Extrusion43" cut sketch "Sketch27" against normal blind 0.5 contours L0 L1 L2 A1 L7 L6 L9 L3 | L2 A1 A0
extrude "Extrusion44" cut sketch "Sketch27" against normal blind 2 contours L14 L15 L16 L17
extrude "Extrusion45" cut sketch "Sketch27" against normal blind 0.5 contours L10 L11 L12 L13
mirror "Mirror1" about plane through (0, 0, 0) normal (0, 0, 1) of "Extrusion45", "Extrusion44", "Extrusion43", "Extrusion42"
sketch "Sketch28" plane through (-10, 26, 30) normal (0, 0, -1) x (-1, 0, 0)
  line L0 (10, 7) -> (-2, 7) projected
  line L1 (-2, 4.5272) -> (-2, 7) projected
  line L2 (0, 4.5272) -> (-2, 4.5272) projected
  line L3 (0, 4.5272) -> (0.3921, 5.0532)
  line L4 (0.3921, 5.0532) -> (0.6381, 5.7636)
  line L5 (0.6381, 5.7636) -> (0.9268, 6.1509)
  line L6 (0.9268, 6.1509) -> (1.0848, 6.6074)
  line L7 (1.0848, 6.6074) -> (1.7585, 6.7277)
  line L8 (1.7585, 6.7277) -> (2.6759, 6.8356)
  line L9 (2.6759, 6.8356) -> (3.1613, 6.6676)
  line L10 (3.1613, 6.6676) -> (4.3741, 6.8842)
  line L11 (4.3741, 6.8842) -> (5.6664, 6.8842)
  line L12 (-10, 0) -> (-10, 7) projected
  line L13 (5.6664, 6.8842) -> (6.5282, 6.9855)
  line L14 (6.5282, 6.9855) -> (8.1832, 6.9349)
  line L15 (8.1832, 6.9349) -> (9.1956, 7)
  point P0 (-10, -26)
  constraints: 24 end point, 4 parallel, 2 perpendicular, 1 point on line
extrude "Extrusion46" cut sketch "Sketch28" against normal blind 2
sketch "Sketch29" plane through (0, 32, 0) normal (0, 1, 0) x (1, 0, 0)
  line L0 (-10, 30) -> (-8, 30) projected
  line L1 (-8, 30) -> (-8, 32) projected
  line L2 (-8, 32) -> (-18, 32) projected
  line L3 (-18, 32) -> (-18, 38) projected
  line L4 (-18, 38) -> (-20, 38) projected
  line L5 (-20, 38) -> (-20, 30) projected
  line L6 (-20, 30) -> (-10, 30) projected
  point P0 (0, 0)
extrude "Extrusion47" add sketch "Sketch29" along normal blind 1
ref_plane "Work Plane2" through (-6.9968, 35.5, 7.1453) normal (0, 1, 0) x (0.7071068, 0, 0.7071068)
split body "Split1" result two bodies by plane through (-6.9968, 35.5, 7.1453) normal (0, 1, 0) first body at (-9.3333, 36, -1.1046)
move or copy body "Move Body1" bodies to move or copy 2 copy no translate (0, 2, 0)
sketch "Sketch30" plane through (-4.1421, 37.5, -10) normal (0, -1, 0) x (1, 0, 0)
  line L0 (0, 0) -> (-5.8579, 5.8579) projected
  line L1 (8.2843, 0) -> (0, 0) projected
  line L2 (14.1421, 5.8579) -> (8.2843, 0) projected
  line L3 (14.1421, 14.1421) -> (14.1421, 5.8579) projected
  line L4 (8.2843, 20) -> (14.1421, 14.1421) projected
  line L5 (0, 20) -> (8.2843, 20) projected
  line L6 (-5.8579, 14.1421) -> (0, 20) projected
  line L7 (-5.8579, 5.8579) -> (-5.8579, 14.1421) projected
  point P0 (4.1421, 10)
extrude "Extrusion48" add sketch "Sketch30" along normal blind 2 bodies 2
sketch "Sketch31" plane through (-10, 26, -30) normal (-1, 0, 0) x (0, 0, 1)
  line L0 (8.0261, 7.8304) -> (6.0082, 8.5) projected
  line L1 (3.2966, 8.5) -> (6.0082, 8.5) projected
  line L2 (3.2966, 8.5) -> (3.0942, 8.0977) projected
  line L3 (3.0942, 8.0977) -> (3.8617, 8.3035)
  line L4 (3.8617, 8.3035) -> (4.5019, 8.2006)
  line L5 (4.5019, 8.2006) -> (5.1184, 8.2912)
  line L6 (5.1184, 8.2912) -> (5.8585, 8.2912)
  line L7 (6.0082, 8.5) -> (3.2966, 8.5) projected
  line L8 (5.8585, 8.2912) -> (6.4566, 8.3512)
  point P0 (30, -26)
  constraints: 10 end point, 1 parallel, 1 point on line
extrude "Extrusion49" cut sketch "Sketch31" against normal blind 10 bodies 3
sketch "Sketch32" plane through (10, 45.5, 4.1421) normal (1, 0, 0) x (0, 0, -1)
  line L0 (22.9194, -16.1432) -> (-8.5151, -16.1432)
  line L1 (-8.5151, -16.1432) -> (-8.5151, 5.9722)
  line L2 (-8.5151, 5.9722) -> (22.9194, 5.9722)
  line L3 (22.9194, 5.9722) -> (22.9194, -16.1432)
  point P0 (4.1421, -45.5)
  constraints: 8 end point, 2 parallel, 1 horizontal, 1 perpendicular
extrude "Extrusion50" cut sketch "Sketch32" along normal blind 10 bodies 2
sketch "Sketch33" plane through (10, 34.5, 4.1421) normal (1, 0, 0) x (0, 0, -1)
  line L0 (-14.3255, 10.1484) -> (21.1289, 10.1484)
  line L1 (21.1289, 10.1484) -> (21.1289, -8.5)
  line L2 (21.1289, -8.5) -> (-14.3255, -8.5)
  line L3 (-14.3255, -8.5) -> (-14.3255, 10.1484)
  point P0 (4.1421, -34.5)
  constraints: 8 end point, 2 parallel, 1 horizontal, 1 perpendicular
extrude "Extrusion51" cut sketch "Sketch33" along normal blind 10 bodies 3
sketch "Sketch34" plane through (-10, 32.6161, -14.375) normal (0, -1, 0) x (1, 0, 0)
  line L0 (0.5, 0) -> (0.5, 3.75) projected
  line L1 (-0.25, 0.9919) -> (0.5, 0.9919)
  line L2 (0.5, 0.9919) -> (0.5, 1.4919)
  line L3 (0.5, 1.4919) -> (-0.25, 1.4919)
  line L4 (-0.25, 1.4919) -> (-0.25, 0.9919)
  line L5 (-0.25, 2.7138) -> (0.5, 2.7138)
  line L6 (0.5, 2.7138) -> (0.5, 3.2138)
  line L7 (0.5, 3.2138) -> (-0.25, 3.2138)
  line L8 (-0.25, 3.2138) -> (-0.25, 2.7138)
  point P0 (10, 14.375)
  point P1 (0.5, 0.9919)
  point P2 (0.5, 2.7138)
  point P3 (0.5, 3.2138)
  dimension "d229" = 0.75
  dimension "d230" = 0
  dimension "d231" = 0.5
  dimension "d232" = 0.5
  constraints: 16 end point, 4 parallel, 2 horizontal, 2 perpendicular, 2 point on line
  measures "d229" distance between parallel lines of L8 L0
  measures "d230" distance between parallel lines of L0 L6
  measures "d231" distance of L7.end L5.start
  measures "d232" distance of L3.end L1.start
extrude "Extrusion52" add sketch "Sketch34" along normal up to surface (4.5 mm away) bodies 3
sketch "Sketch35" plane through (-10, 32.6161, -13.3831) normal (0, 0, -1) x (-1, 0, 0)
  line L0 (0, -3.2858) -> (0.8056, -3.2858)
  line L1 (0.8056, -3.2858) -> (0.8056, -2.7858)
  line L2 (0.8056, -2.7858) -> (0, -2.7858)
  line L3 (0, -2.7858) -> (0, -3.2858)
  line L4 (0, 0) -> (0, -4.5) projected
  line L5 (0, -1.3) -> (0.8056, -1.3)
  line L6 (0.8056, -1.3) -> (0.8056, -0.8)
  line L7 (0.8056, -0.8) -> (0, -0.8)
  line L8 (0, -0.8) -> (0, -1.3)
  point P0 (-10, -32.6161)
  point P1 (0, -0.8)
  dimension "d233" = 0.5
  dimension "d234" = 0.5
  dimension "d235" = 0.8
  constraints: 16 end point, 4 parallel, 2 horizontal, 2 perpendicular, 2 point on line
  measures "d233" distance of L5.end L6.end
  measures "d234" distance of L0.end L1.end
  measures "d235" distance from line of L4.start L7
extrude "Extrusion53" add sketch "Sketch35" along normal blind 2 and the other way blind 4 bodies 3
sketch "Sketch36" plane through (-10, 26, -30) normal (-1, 0, 0) x (0, 0, 1)
  line L0 (3.125, 6.6161) -> (6.875, 6.6161) projected
  line L1 (3.125, 6.6161) -> (6.875, 6.6161) projected
  line L2 (3.125, 2.1161) -> (3.125, 6.6161) projected
  arc A0 (6.875, 6.6161) -> (3.125, 6.6161) centre (5, 2.229) ccw
  line L3 (-8, 7) -> (23.8579, 7) projected
  point P0 (30, -26)
  constraints: 2 point on circle, 1 centre point, 1 tangent
extrude "Extrusion54" cut sketch "Sketch36" against normal blind 0.5 bodies 3
pattern_linear "Rectangular Pattern8" count 5 spacing 12.5 along (0, 0, 1) count 2 spacing 14 along (0, -1, 0) of "Extrusion54" bodies 3
extrude "Extrusion55" add sketch "Sketch34" against normal up to surface (0.3839 mm away) bodies 3
body "Solid2"
body "Solid3"
